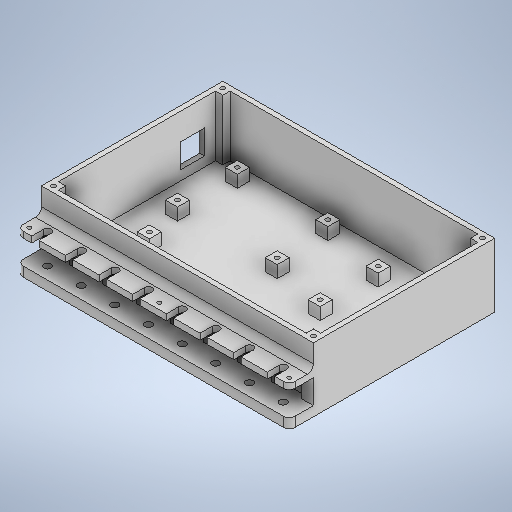
# Autodesk Inventor part: ebox
Saved by Autodesk Inventor 2025.2 (Build 292293000, 293)
## iProperties
Created: 2025-01-01
Part Number: ebox
Material: Generic
Document SubType Name: Modeling
Designer: email
Density: 1 g/cm^3
Appearance: Default
Author: email
Autodesk Inventor part; units mm, degrees
ref_plane "YZ Plane" through (0, 0, 0) normal (1, 0, 0) x (0, 1, 0)
ref_plane "XZ Plane" through (0, 0, 0) normal (0, 1, 0) x (-1, 0, 0)
ref_plane "XY Plane" through (0, 0, 0) normal (0, 0, 1) x (1, 0, 0)
sketch "Sketch1" plane through (0, 0, 0) normal (0, 1, 0) x (-1, 0, 0)
  line L0 (0, 0) -> (-225, 0)
  line L1 (-225, 0) -> (-225, -150)
  line L2 (-225, -150) -> (0, -150)
  line L3 (0, -150) -> (0, 0)
  line L4 (-12.5, -136.845) -> (-114.1, -136.845)
  line L5 (-114.1, -136.845) -> (-114.1, -83.505)
  line L6 (-114.1, -83.505) -> (-12.5, -83.505)
  line L7 (-12.5, -83.505) -> (-12.5, -136.845)
  line L8 (-4, -4) -> (-221, -4)
  line L9 (-221, -4) -> (-221, -146)
  line L10 (-221, -146) -> (-4, -146)
  line L11 (-4, -146) -> (-4, -4)
  line L12 (-153.3391, -125.2346) -> (-208.3391, -125.2346)
  line L13 (-208.3391, -125.2346) -> (-208.3391, -70.2346)
  line L14 (-208.3391, -70.2346) -> (-153.3391, -70.2346)
  line L15 (-153.3391, -70.2346) -> (-153.3391, -125.2346)
  line L16 (-12.6469, -54.1694) -> (-42.6469, -54.1694)
  line L17 (-42.6469, -54.1694) -> (-42.6469, -34.1694)
  line L18 (-42.6469, -34.1694) -> (-12.6469, -34.1694)
  line L19 (-12.6469, -34.1694) -> (-12.6469, -54.1694)
  line L20 (-15.41, -128.945) -> (-4, -128.945)
  line L21 (-4, -128.945) -> (-4, -117.045)
  line L22 (-4, -117.045) -> (-15.41, -117.045)
  line L23 (-15.41, -117.045) -> (-15.41, -128.945)
  circle A0 centre (-27.74, -134.305) radius 1.75
  circle A1 centre (-26.47, -86.045) radius 1.75
  circle A2 centre (-102.67, -134.305) radius 1.75
  circle A3 centre (-109.02, -86.045) radius 1.75
  circle A4 centre (-156.8391, -121.7346) radius 1.75
  circle A5 centre (-204.8391, -121.7346) radius 1.75
  circle A6 centre (-156.8391, -73.7346) radius 1.75
  circle A7 centre (-204.8391, -73.7346) radius 1.75
  circle A8 centre (-37.5669, -51.6294) radius 1.75
  circle A9 centre (-37.5669, -36.7094) radius 1.75
  line L24 (-22.74, -139.305) -> (-32.74, -139.305)
  line L25 (-32.74, -139.305) -> (-32.74, -129.305)
  line L26 (-32.74, -129.305) -> (-22.74, -129.305)
  line L27 (-22.74, -129.305) -> (-22.74, -139.305)
  line L28 (-22.74, -139.305) -> (-32.74, -129.305) construction
  line L29 (-32.74, -139.305) -> (-22.74, -129.305) construction
  line L30 (-21.47, -81.045) -> (-31.47, -81.045)
  line L31 (-31.47, -81.045) -> (-31.47, -91.045)
  line L32 (-31.47, -91.045) -> (-21.47, -91.045)
  line L33 (-21.47, -91.045) -> (-21.47, -81.045)
  line L34 (-21.47, -81.045) -> (-31.47, -91.045) construction
  line L35 (-31.47, -81.045) -> (-21.47, -91.045) construction
  line L36 (-114.02, -81.045) -> (-104.02, -81.045)
  line L37 (-104.02, -81.045) -> (-104.02, -91.045)
  line L38 (-104.02, -91.045) -> (-114.02, -91.045)
  line L39 (-114.02, -91.045) -> (-114.02, -81.045)
  line L40 (-114.02, -81.045) -> (-104.02, -91.045) construction
  line L41 (-104.02, -81.045) -> (-114.02, -91.045) construction
  line L42 (-107.67, -139.305) -> (-97.67, -139.305)
  line L43 (-97.67, -139.305) -> (-97.67, -129.305)
  line L44 (-97.67, -129.305) -> (-107.67, -129.305)
  line L45 (-107.67, -129.305) -> (-107.67, -139.305)
  line L46 (-107.67, -139.305) -> (-97.67, -129.305) construction
  line L47 (-97.67, -139.305) -> (-107.67, -129.305) construction
  line L48 (-151.8391, -126.7346) -> (-161.8391, -126.7346)
  line L49 (-161.8391, -126.7346) -> (-161.8391, -116.7346)
  line L50 (-161.8391, -116.7346) -> (-151.8391, -116.7346)
  line L51 (-151.8391, -116.7346) -> (-151.8391, -126.7346)
  line L52 (-151.8391, -126.7346) -> (-161.8391, -116.7346) construction
  line L53 (-161.8391, -126.7346) -> (-151.8391, -116.7346) construction
  line L54 (-209.8391, -126.7346) -> (-199.8391, -126.7346)
  line L55 (-199.8391, -126.7346) -> (-199.8391, -116.7346)
  line L56 (-199.8391, -116.7346) -> (-209.8391, -116.7346)
  line L57 (-209.8391, -116.7346) -> (-209.8391, -126.7346)
  line L58 (-209.8391, -126.7346) -> (-199.8391, -116.7346) construction
  line L59 (-199.8391, -126.7346) -> (-209.8391, -116.7346) construction
  line L60 (-209.8391, -68.7346) -> (-199.8391, -68.7346)
  line L61 (-199.8391, -68.7346) -> (-199.8391, -78.7346)
  line L62 (-199.8391, -78.7346) -> (-209.8391, -78.7346)
  line L63 (-209.8391, -78.7346) -> (-209.8391, -68.7346)
  line L64 (-209.8391, -68.7346) -> (-199.8391, -78.7346) construction
  line L65 (-199.8391, -68.7346) -> (-209.8391, -78.7346) construction
  line L66 (-161.8391, -68.7346) -> (-151.8391, -68.7346)
  line L67 (-151.8391, -68.7346) -> (-151.8391, -78.7346)
  line L68 (-151.8391, -78.7346) -> (-161.8391, -78.7346)
  line L69 (-161.8391, -78.7346) -> (-161.8391, -68.7346)
  line L70 (-161.8391, -68.7346) -> (-151.8391, -78.7346) construction
  line L71 (-151.8391, -68.7346) -> (-161.8391, -78.7346) construction
  line L72 (-42.5669, -46.6294) -> (-32.5669, -46.6294)
  line L73 (-32.5669, -46.6294) -> (-32.5669, -56.6294)
  line L74 (-32.5669, -56.6294) -> (-42.5669, -56.6294)
  line L75 (-42.5669, -56.6294) -> (-42.5669, -46.6294)
  line L76 (-42.5669, -46.6294) -> (-32.5669, -56.6294) construction
  line L77 (-32.5669, -46.6294) -> (-42.5669, -56.6294) construction
  line L78 (-32.5669, -41.7094) -> (-42.5669, -41.7094)
  line L79 (-42.5669, -41.7094) -> (-42.5669, -31.7094)
  line L80 (-42.5669, -31.7094) -> (-32.5669, -31.7094)
  line L81 (-32.5669, -31.7094) -> (-32.5669, -41.7094)
  line L82 (-32.5669, -41.7094) -> (-42.5669, -31.7094) construction
  line L83 (-42.5669, -41.7094) -> (-32.5669, -31.7094) construction
  line L84 (0, -4) -> (-225, -4)
  line L85 (-225, -4) -> (-225, 20)
  line L86 (-225, 20) -> (0, 20)
  line L87 (0, 20) -> (0, -4)
  circle A10 centre (-15, 10) radius 2.95
  circle A11 centre (-42.85, 10) radius 2.95
  circle A12 centre (-70.7, 10) radius 2.95
  circle A13 centre (-98.55, 10) radius 2.95
  circle A14 centre (-126.4, 10) radius 2.95
  circle A15 centre (-154.25, 10) radius 2.95
  circle A16 centre (-182.1, 10) radius 2.95
  circle A17 centre (-209.95, 10) radius 2.95
  point P0 (-156.8391, -73.7346)
  point P1 (-225, 8)
  dimension "d0" = 225
  dimension "d1" = 150
  dimension "d2" = 101.6
  dimension "d3" = 53.34
  dimension "d5" = 4
  dimension "d6" = 217
  dimension "d7" = 142
  dimension "d8" = 4
  dimension "d9" = 8.5
  dimension "d10" = 55
  dimension "d11" = 55
  dimension "d12" = 30
  dimension "d13" = 20
  dimension "d14" = 7.9
  dimension "d15" = 8.5
  dimension "d16" = 11.9
  dimension "d17" = 2.54
  dimension "d18" = 3.5
  dimension "d19" = 15.24
  dimension "d20" = 3.5
  dimension "d21" = 3.5
  dimension "d22" = 3.5
  dimension "d23" = 2.54
  dimension "d24" = 13.97
  dimension "d26" = 2.54
  dimension "d27" = 90.17
  dimension "d28" = 2.54
  dimension "d29" = 96.52
  dimension "d30" = 3.5
  dimension "d31" = 3.5
  dimension "d32" = 3.5
  dimension "d33" = 3.5
  dimension "d34" = 3.5
  dimension "d35" = 3.5
  dimension "d36" = 3.5
  dimension "d38" = 3.5
  dimension "d39" = 3.5
  dimension "d40" = 3.5
  dimension "d41" = 3.5
  dimension "d42" = 3.5
  dimension "d43" = 3.5
  dimension "d44" = 2.54
  dimension "d45" = 5.08
  dimension "d46" = 5.08
  dimension "d47" = 2.54
  dimension "d54" = 10
  dimension "d55" = 10
  dimension "d56" = 10
  dimension "d57" = 10
  dimension "d58" = 10
  dimension "d59" = 10
  dimension "d60" = 10
  dimension "d61" = 10
  dimension "d65" = 10
  dimension "d66" = 10
  dimension "d67" = 10
  dimension "d68" = 10
  dimension "d69" = 10
  dimension "d70" = 10
  dimension "d71" = 10
  dimension "d72" = 10
  dimension "d73" = 10
  dimension "d74" = 10
  dimension "d75" = 10
  constraints: 176 end point, 34 parallel, 22 midpoint, 18 centre point, 18 horizontal, 17 perpendicular, 2 point on line, 14 other
  measures "d0" distance of L1.end L2.end
  measures "d1" distance of L0.end L1.end
  measures "d2" distance of L4.start L4.end
  measures "d3" distance of L4.end L5.end
  measures "d5" distance between parallel lines of L0 L8
  measures "d6" distance of L9.end L10.end
  measures "d7" distance of L8.end L9.end
  measures "d8" distance between parallel lines of L3 L11
  measures "d9" distance between parallel lines of L11 L7
  measures "d10" distance of L12.end L13.end
  measures "d11" distance of L13.end L14.end
  measures "d12" distance of L16.start L16.end
  measures "d13" distance of L16.end L17.end
  measures "d14" distance between parallel lines of L4 L20
  measures "d15" distance between parallel lines of L7 L21
  measures "d16" distance of L22.end L20.start
  measures "d17" distance from line of L4 A0.centre
  measures "d18" diameter of A0
  measures "d19" distance from line of L7 A0.centre
  measures "d20" diameter of A1
  measures "d21" diameter of A3
  measures "d22" diameter of A2
  measures "d23" distance from line of L6 A1.centre
  measures "d24" distance from line of L7 A1.centre
  measures "d26" distance from line of L4 A2.centre
  measures "d27" distance from line of A2.centre L7
  measures "d28" distance from line of L6 A3.centre
  measures "d29" distance from line of L7 A3.centre
  measures "d30" diameter of A4
  measures "d31" diameter of A5
  measures "d32" diameter of A6
  measures "d33" diameter of A7
  measures "d34" distance from line of L12 A4.centre
  measures "d35" distance from line of L15 A4.centre
  measures "d36" distance from line of L14 A6.centre
  measures "d38" distance from line of L13 A7.centre
  measures "d39" distance from line of L14 A7.centre
  measures "d40" distance from line of L13 A5.centre
  measures "d41" distance from line of L12 A5.centre
  measures "d42" diameter of A8
  measures "d43" diameter of A9
  measures "d44" distance from line of L16 A8.centre
  measures "d45" distance from line of L17 A8.centre
  measures "d46" distance from line of L17 A9.centre
  measures "d47" distance from line of L18 A9.centre
  measures "d54" distance of L24.end L25.end
  measures "d55" distance of L25.end L26.end
  measures "d56" distance of L42.end L43.end
  measures "d57" distance of L43.end L44.end
  measures "d58" distance of L31.end L32.end
  measures "d59" distance of L30.end L31.end
  measures "d60" distance of L37.end L38.end
  measures "d61" distance of L36.end L37.end
  measures "d65" distance of L48.end L49.end
  measures "d66" distance of L49.end L50.end
  measures "d67" distance of L54.end L55.end
  measures "d68" distance of L55.end L56.end
  measures "d69" distance of L66.end L67.end
  measures "d70" distance of L66.start L66.end
  measures "d71" distance of L62.end L60.start
  measures "d72" distance of L60.start L60.end
  measures "d73" distance of L73.end L74.end
  measures "d74" distance of L72.end L73.end
  measures "d75" distance of L78.start L78.end
extrude "Extrusion1" add sketch "Sketch1" against normal blind 3 contours L3 L84 L8 L1 L0 | L3 L2 L1 L84 L9 L10 L11 | L11 L22 L7 L6 L33 L30 L31 L37 L36 L39 L5 L4 L45 L42 L43 L25 L24 L27 L20 L10 L9 L8 | L11 L20 L7 L22 | L22 L23 L20 L7 L4 L27 L26 L25 L43 L44 L45 L5 L6 L39 L38 L37 L31 L32 L33 | L7 L20 L23 L22 | L33 L32 L31 L6 | L6 L31 L30 L33 | L27 L24 L25 L4 | L4 L25 L26 L27 | L37 L38 L39 L6 | L6 L39 L36 L37 | L43 L42 L45 L4 | L4 L45 L44 L43 | L15 L50 L51 L48 L49 L12 | L12 L49 L50 L15 | L12 L55 L56 L13 L62 L61 L14 L69 L68 L15 L50 L49 | L55 L54 L57 L56 L13 L12 | L12 L13 L56 L55 | L68 L69 L14 L15 | L15 L14 L69 L66 L67 L68 | L62 L63 L60 L61 L14 L13 | L13 L14 L61 L62 | L16 L73 L72 L75 L17 L18 L79 L78 L81 L19 | L73 L74 L75 L16 | L16 L75 L72 L73 | L81 L78 L79 L18 | L18 L79 L80 L81 | A0 | A1 | A2 | A3 | A4 | A5 | A6 | A7 | A8 | A9
extrude "Extrusion2" add sketch "Sketch1" along normal blind 50 contours L3 L84 L8 L1 L0 | L3 L2 L1 L84 L9 L10 L11
extrude "Extrusion3" add sketch "Sketch1" along normal blind 10 contours L33 L32 L31 L6 | L6 L31 L30 L33 | L27 L24 L25 L4 | L4 L25 L26 L27 | L37 L38 L39 L6 | L6 L39 L36 L37 | L43 L42 L45 L4 | L4 L45 L44 L43 | L15 L50 L51 L48 L49 L12 | L12 L49 L50 L15 | L55 L54 L57 L56 L13 L12 | L12 L13 L56 L55 | L68 L69 L14 L15 | L15 L14 L69 L66 L67 L68 | L62 L63 L60 L61 L14 L13 | L13 L14 L61 L62 | L73 L74 L75 L16 | L16 L75 L72 L73 | L81 L78 L79 L18 | L18 L79 L80 L81
extrude "Extrusion4" add sketch "Sketch1" along normal blind 5 and the other way blind 3 contours L0 L85 L86 L87
sketch "Sketch2" plane through (0, 50, 0) normal (0, 0, 1) x (1, 0, 0)
  line L0 (7, -25) -> (23, -25)
  line L1 (23, -25) -> (23, -45)
  line L2 (23, -45) -> (7, -45)
  line L3 (7, -45) -> (7, -25)
  line L4 (7, -25) -> (23, -45) construction
  line L5 (23, -25) -> (7, -45) construction
  line L6 (34.85, -25) -> (50.85, -25)
  line L7 (50.85, -25) -> (50.85, -45)
  line L8 (50.85, -45) -> (34.85, -45)
  line L9 (34.85, -45) -> (34.85, -25)
  line L10 (34.85, -25) -> (50.85, -45) construction
  line L11 (50.85, -25) -> (34.85, -45) construction
  line L12 (62.7, -25) -> (78.7, -25)
  line L13 (78.7, -25) -> (78.7, -45)
  line L14 (78.7, -45) -> (62.7, -45)
  line L15 (62.7, -45) -> (62.7, -25)
  line L16 (62.7, -25) -> (78.7, -45) construction
  line L17 (78.7, -25) -> (62.7, -45) construction
  line L18 (90.55, -25) -> (106.55, -25)
  line L19 (106.55, -25) -> (106.55, -45)
  line L20 (106.55, -45) -> (90.55, -45)
  line L21 (90.55, -45) -> (90.55, -25)
  line L22 (90.55, -25) -> (106.55, -45) construction
  line L23 (106.55, -25) -> (90.55, -45) construction
  line L24 (118.4, -25) -> (134.4, -25)
  line L25 (134.4, -25) -> (134.4, -45)
  line L26 (134.4, -45) -> (118.4, -45)
  line L27 (118.4, -45) -> (118.4, -25)
  line L28 (118.4, -25) -> (134.4, -45) construction
  line L29 (134.4, -25) -> (118.4, -45) construction
  line L30 (146.25, -25) -> (162.25, -25)
  line L31 (162.25, -25) -> (162.25, -45)
  line L32 (162.25, -45) -> (146.25, -45)
  line L33 (146.25, -45) -> (146.25, -25)
  line L34 (146.25, -25) -> (162.25, -45) construction
  line L35 (162.25, -25) -> (146.25, -45) construction
  line L36 (174.1, -25) -> (190.1, -25)
  line L37 (190.1, -25) -> (190.1, -45)
  line L38 (190.1, -45) -> (174.1, -45)
  line L39 (174.1, -45) -> (174.1, -25)
  line L40 (174.1, -25) -> (190.1, -45) construction
  line L41 (190.1, -25) -> (174.1, -45) construction
  line L42 (201.95, -25) -> (217.95, -25)
  line L43 (217.95, -25) -> (217.95, -45)
  line L44 (217.95, -45) -> (201.95, -45)
  line L45 (201.95, -45) -> (201.95, -25)
  line L46 (201.95, -25) -> (217.95, -45) construction
  line L47 (217.95, -25) -> (201.95, -45) construction
  line L48 (0, -45) -> (0, 0) projected
  line L49 (0, -45) -> (225, -45) projected
  point P0 (15, -35)
  point P1 (42.85, -35)
  point P2 (70.7, -35)
  point P3 (98.55, -35)
  point P4 (126.4, -35)
  point P5 (154.25, -35)
  point P6 (182.1, -35)
  point P7 (209.95, -35)
  dimension "d105" = 16
  dimension "d106" = 20
  dimension "d109" = 27.85
  dimension "d132" = 15
  dimension "d133" = 10
  constraints: 96 end point, 16 midpoint, 2 horizontal, 2 parallel, 1 collinear, 1 perpendicular, 76 other
  measures "d105" distance of L0.start L0.end
  measures "d106" distance of L2.end L0.start
  measures "d109" distance of L0.start L6.start
  measures "d132" distance from line of L48 point (15, -35)
  measures "d133" distance from line of L49 point (15, -35)
extrude "Extrusion5" cut sketch "Sketch2" against normal blind 4
ref_plane "Work Plane1" through (0, 25, 0) normal (0, 1, 0) x (1, 0, 0)
sketch "Sketch3" plane through (0, 25, 0) normal (0, 1, 0) x (1, 0, 0)
  line L0 (0, 150) -> (0, 0) projected
  line L1 (0, 0) -> (225, 0)
  line L2 (225, 0) -> (225, -20)
  line L3 (225, -20) -> (0, -20)
  line L4 (0, -20) -> (0, 0)
  circle A0 centre (15, -10) radius 2.95 construction
  line L5 (11.95, -10) -> (11.95, -20)
  line L6 (18.05, -9.9879) -> (18.05, -20)
  arc A1 (18.05, -9.9879) -> (11.95, -10) centre (15, -10) ccw
  line L7 (11.95, -20) -> (18.05, -20)
  line L8 (39.8, -10) -> (39.8, -20)
  line L9 (45.9, -9.9879) -> (45.9, -20)
  arc A2 (45.9, -9.9879) -> (39.8, -10) centre (42.85, -10) ccw
  line L10 (39.8, -20) -> (45.9, -20)
  line L11 (67.65, -10) -> (67.65, -20)
  line L12 (73.75, -9.9879) -> (73.75, -20)
  arc A3 (73.75, -9.9879) -> (67.65, -10) centre (70.7, -10) ccw
  line L13 (67.65, -20) -> (73.75, -20)
  line L14 (95.5, -10) -> (95.5, -20)
  line L15 (101.6, -9.9879) -> (101.6, -20)
  arc A4 (101.6, -9.9879) -> (95.5, -10) centre (98.55, -10) ccw
  line L16 (95.5, -20) -> (101.6, -20)
  line L17 (123.35, -10) -> (123.35, -20)
  line L18 (129.45, -9.9879) -> (129.45, -20)
  arc A5 (129.45, -9.9879) -> (123.35, -10) centre (126.4, -10) ccw
  line L19 (123.35, -20) -> (129.45, -20)
  line L20 (151.2, -10) -> (151.2, -20)
  line L21 (157.3, -9.9879) -> (157.3, -20)
  arc A6 (157.3, -9.9879) -> (151.2, -10) centre (154.25, -10) ccw
  line L22 (151.2, -20) -> (157.3, -20)
  line L23 (179.05, -10) -> (179.05, -20)
  line L24 (185.15, -9.9879) -> (185.15, -20)
  arc A7 (185.15, -9.9879) -> (179.05, -10) centre (182.1, -10) ccw
  line L25 (179.05, -20) -> (185.15, -20)
  line L26 (206.9, -10) -> (206.9, -20)
  line L27 (213, -9.9879) -> (213, -20)
  arc A8 (213, -9.9879) -> (206.9, -10) centre (209.95, -10) ccw
  line L28 (206.9, -20) -> (213, -20)
  circle A9 centre (5, -15) radius 1.5
  circle A10 centre (220, -15) radius 1.5
  circle A11 centre (112.5, -15) radius 1.5
  point P0 (18.125, -20)
  point P1 (45.975, -20)
  point P2 (73.825, -20)
  point P3 (101.675, -20)
  point P4 (129.525, -20)
  point P5 (157.375, -20)
  point P6 (185.225, -20)
  point P7 (213.075, -20)
  point P8 (112.5, -20)
  dimension "d118" = 20
  dimension "d119" = 225
  dimension "d140" = 27.85
  dimension "d145" = 3.05
  dimension "d146" = 3
  dimension "d147" = 5
  dimension "d148" = 5
  dimension "d149" = 3
  dimension "d150" = 5
  dimension "d151" = 5
  dimension "d152" = 3
  dimension "d153" = 5
  constraints: 54 end point, 49 horizontal alignment, 16 point on circle, 15 parallel, 11 centre point, 7 collinear, 7 equal radius, 3 horizontal, 2 vertical, 1 coincident, 1 perpendicular, 1 tangent, 7 other
  measures "d118" distance of L1.end L2.end
  measures "d119" distance of L2.end L4.start
  measures "d140" distance of A0.centre point (42.85, -10)
  measures "d145" radius of A1
  measures "d146" diameter of A9
  measures "d147" distance from line of L4 A9.centre
  measures "d149" diameter of A10
  measures "d150" distance from line of L2 A10.centre
  measures "d152" diameter of A11
  measures "d153" distance of point (112.5, -20) A11.centre
extrude "Extrusion6" add sketch "Sketch3" along normal blind 5 contours L1 L2 L3 L27 A8 L26 L24 A7 L23 L21 A6 L20 L18 A5 L17 L15 A4 L14 L12 A3 L11 L9 A2 L8 L6 A1 L5 L4
fillet "Fillet2" radius 5 4 edges at (0, 27.5, 20) (0, 1, 20) (225, 27.5, 20) (225, 1, 20)
fillet "Fillet3" radius 5 1 edges at (112.5, 30, 0)
sketch "Sketch4" plane through (0, 50, 0) normal (0, 1, 0) x (1, 0, 0)
  line L0 (0, 0) -> (10, 0)
  line L1 (10, 0) -> (10, 10)
  line L2 (10, 10) -> (0, 10)
  line L3 (0, 10) -> (0, 0)
  circle A0 centre (5, 5) radius 1.75
  line L4 (0, -15) -> (0, 150) projected
  line L5 (0, 150) -> (10, 150)
  line L6 (10, 150) -> (10, 140)
  line L7 (10, 140) -> (0, 140)
  line L8 (0, 140) -> (0, 150)
  circle A1 centre (5, 145) radius 1.75
  line L9 (0, 150) -> (225, 150) projected
  line L10 (225, 150) -> (215, 150)
  line L11 (215, 150) -> (215, 140)
  line L12 (215, 140) -> (225, 140)
  line L13 (225, 140) -> (225, 150)
  line L14 (7, 0) -> (23, 0) projected
  line L15 (225, 0) -> (215, 0)
  line L16 (215, 0) -> (215, 10)
  line L17 (215, 10) -> (225, 10)
  line L18 (225, 10) -> (225, 0)
  circle A2 centre (220, 145) radius 1.75
  circle A3 centre (220, 5) radius 1.75
  point P0 (5, 10)
  point P1 (5, 140)
  point P2 (10, 145)
  point P3 (217.95, 0)
  point P4 (215, 145)
  point P5 (220, 140)
  point P6 (217.95, 0)
  point P7 (215, 5)
  dimension "d154" = 10
  dimension "d155" = 10
  dimension "d156" = 3.5
  dimension "d157" = 5
  dimension "d158" = 5
  dimension "d159" = 10
  dimension "d160" = 10
  dimension "d161" = 3.5
  dimension "d162" = 5
  dimension "d163" = 5
  dimension "d164" = 10
  dimension "d165" = 10
  dimension "d166" = 3.5
  dimension "d167" = 5
  dimension "d168" = 5
  dimension "d169" = 10
  dimension "d170" = 10
  dimension "d171" = 3.5
  dimension "d182" = 5
  dimension "d183" = 5
  constraints: 32 end point, 11 equal length, 6 midpoint, 4 centre point, 4 horizontal, 4 perpendicular
  measures "d154" distance of L1.end L2.end
  measures "d155" distance of L0.end L1.end
  measures "d156" diameter of A0
  measures "d157" distance of point (5, 10) A0.centre
  measures "d158" distance from line of L1 A0.centre
  measures "d159" distance of L5.end L6.end
  measures "d160" distance of L6.end L7.end
  measures "d161" diameter of A1
  measures "d162" distance of point (5, 140) A1.centre
  measures "d163" distance of point (10, 145) A1.centre
  measures "d164" distance of L10.end L11.end
  measures "d165" distance of L11.end L12.end
  measures "d166" diameter of A2
  measures "d167" distance of point (215, 145) A2.centre
  measures "d168" distance of point (220, 140) A2.centre
  measures "d169" distance of L16.end L17.end
  measures "d170" distance of L15.end L16.end
  measures "d171" diameter of A3
  measures "d182" distance from line of L17 A3.centre
  measures "d183" distance of point (215, 5) A3.centre
extrude "Extrusion7" add sketch "Sketch4" against normal up to surface (50 mm away) contours L3 L2 L1 L0 | A0 | L4 L5 L6 L7 | A1 | L9 L13 L12 L11 | L15 L16 L17 L18 | A2 | A3
extrude "Extrusion8" cut sketch "Sketch4" against normal blind 10 contours A0 | A1 | A2 | A3
sketch "Sketch5" plane through (0, -3, -150) normal (-1, 0, 0) x (0, 0, 1)
  line L0 (19, 31) -> (39, 31)
  line L1 (39, 31) -> (39, 11)
  line L2 (39, 11) -> (19, 11)
  line L3 (19, 11) -> (19, 31)
  line L4 (10, 3) -> (140, 3) projected
  line L5 (4, 3) -> (4, 43)
  point P0 (150, 3)
  dimension "d176" = 20
  dimension "d177" = 20
  dimension "d180" = 8
  dimension "d181" = 15
  constraints: 10 end point, 2 parallel, 1 horizontal, 1 perpendicular
  measures "d176" distance of L0.start L0.end
  measures "d177" distance of L2.end L0.start
  measures "d180" distance between parallel lines of L4 L2
  measures "d181" distance between parallel lines of L5 L3
extrude "Extrusion9" cut sketch "Sketch5" against normal up to surface (4 mm away)
body "Solid1"
